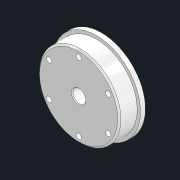
# Autodesk Inventor part: base3
Saved by Autodesk Inventor 2021 (Build 250183000, 183)
## iProperties
Created: 2021-07-17
Part Number: base3
Material: ABS プラスチック
Document SubType Name: Modeling
Designer: yuta0
Density: 1.06 g/cm^3
Appearance: 滑らか - 白
Author: yuta0
Autodesk Inventor part; units mm, degrees
ref_plane "YZ Plane" through (0, 0, 0) normal (1, 0, 0) x (0, 1, 0)
ref_plane "XZ Plane" through (0, 0, 0) normal (0, 1, 0) x (-1, 0, 0)
ref_plane "XY Plane" through (0, 0, 0) normal (0, 0, 1) x (1, 0, 0)
sketch "スケッチ1" plane through (0, 0, 0) normal (1, 0, 0) x (0, 1, 0)
  line L0 (7, 0) -> (7, 0)
  line L1 (0, -9) -> (0, -14)
  line L2 (0, -14) -> (27, -14)
  line L3 (27, -14) -> (27, -11)
  line L4 (27, -11) -> (25, -11)
  line L5 (25, -11) -> (25, 0)
  line L6 (25, 0) -> (7, 0)
  line L7 (7, 0) -> (4, 0)
  line L8 (4, 0) -> (4, -9)
  line L9 (4, -9) -> (0, -9)
  point P0 (0, 0)
  dimension "d2" = 11
  dimension "d3" = 3
  dimension "d4" = 25
  dimension "d5" = 2
  dimension "d35" = 0
  dimension "d36" = 7
  dimension "d37" = 4
  dimension "d45" = 9
  constraints: 21 end point, 7 perpendicular, 1 horizontal, 1 horizontal alignment, 1 vertical, 1 vertical alignment
  measures "d2" distance of L4.end L5.end
  measures "d3" distance of L2.end L3.end
  measures "d4" distance from line of point (0, 0) L5
  measures "d5" distance of L3.end L4.end
  measures "d35" distance of L0.start L0.end
  measures "d36" distance between parallel lines of L1 L0
  measures "d37" distance of L8.end L1.start
  measures "d45" distance from line of point (0, 0) L9
revolve "回転1" add sketch "スケッチ1" angle 360 about axis through (0, 0, -9) along (0, 0, -1)
chamfer "面取り1" distance 1 angle 45 1 edges at (0, -25, 0)
sketch "スケッチ2" plane through (0, 0, -14) normal (0, 0, -1) x (-1, 0, 0)
  point P0 (0, 0)
hole "穴1" at (0, 0, -14) direction (0, 0, 1) diameter 4.5 end through all clearance for "Socket Head Cap Screw" size "M4" standard "Ansi Metric M Profile"
sketch "スケッチ3" plane through (0, 0, -14) normal (0, 0, -1) x (-1, 0, 0)
  circle A0 centre (0, 0) radius 21
  point P0 (0, 0)
  point P1 (0, -21)
  point P2 (18.1865, -10.5)
  point P3 (18.1865, 10.5)
  point P4 (0, 21)
  point P5 (-18.1865, 10.5)
  point P6 (-18.1865, -10.5)
  dimension "d20" = 42
  dimension "d23" = 360
  constraints: 1 coincident, 1 vertical alignment, 9 other
hole "穴2" at (0, -21, -14) at (-18.1865, -10.5, -14) at (-18.1865, 10.5, -14) at (0, 21, -14) at (18.1865, 10.5, -14) at (18.1865, -10.5, -14) direction (0, 0, 1) diameter 3.2 end through all clearance for "Socket Head Cap Screw" size "M3" standard "Ansi Metric M Profile"
chamfer "面取り4" distance 0.5 angle 45 1 edges at (0, -4, 0)
